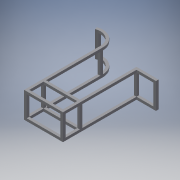
# Autodesk Inventor part: Frame
Saved by Autodesk Inventor 2017 (Build 210142000, 142)
## iProperties
Created: 2017-02-13
Part Number: Frame
Material: Generic
Document SubType Name: Modeling
Designer: Koen
Density: 1 g/cm^3
Appearance: Default
Author: Koen
Autodesk Inventor part; units mm, degrees
ref_plane "YZ Plane" through (0, 0, 0) normal (1, 0, 0) x (0, 1, 0)
ref_plane "XZ Plane" through (0, 0, 0) normal (0, 1, 0) x (-1, 0, 0)
ref_plane "XY Plane" through (0, 0, 0) normal (0, 0, 1) x (1, 0, 0)
sketch "Sketch1" plane through (0, 0, 0) normal (0, 0, 1) x (1, 0, 0)
  line L0 (-300, 150) -> (300, 150)
  line L1 (300, 150) -> (300, -150)
  line L2 (300, -150) -> (-300, -150)
  line L3 (-300, -150) -> (-300, 150)
  line L4 (-300, 150) -> (-260, 150)
  line L5 (-260, 150) -> (-260, 1026.7461)
  line L6 (-260, 1026.7461) -> (-300, 1026.7461)
  line L7 (-300, 1026.7461) -> (-300, 150)
  line L8 (300, 150) -> (260, 150)
  line L9 (260, 150) -> (260, 1026.7461)
  line L10 (260, 1026.7461) -> (300, 1026.7461)
  line L11 (300, 1026.7461) -> (300, 150)
  line L12 (300, 1026.7461) -> (600, 1026.7461)
  line L13 (600, 1026.7461) -> (600, 986.7461)
  line L14 (600, 986.7461) -> (300, 986.7461)
  line L15 (300, 986.7461) -> (300, 1026.7461)
  line L16 (-260, 110) -> (260, 110)
  line L17 (260, 110) -> (260, -110)
  line L18 (260, -110) -> (-260, -110)
  line L19 (-260, -110) -> (-260, 110)
  arc A0 (-260, 1026.7461) -> (-578.8395, 1250) centre (-497.5818, 1026.7461) ccw
  arc A1 (-300, 1026.7461) -> (-565.1587, 1212.4123) centre (-497.5818, 1026.7461) ccw
  line L20 (-565.1587, 1212.4123) -> (-578.8395, 1250)
  point P0 (0, 0)
  point P1 (0, 110)
  point P2 (-260, 0)
  dimension "d0" = 40
  dimension "d1" = 40
  dimension "d2" = 40
  dimension "d3" = 40
  dimension "d4" = 40
  dimension "d6" = 600
  dimension "d7" = 1400
  dimension "d8" = 1136.7461
  dimension "d9" = 300
  dimension "d10" = 300
  dimension "d11" = 110
  constraints: 42 end point, 9 parallel, 6 horizontal, 5 perpendicular, 4 point on circle, 3 vertical alignment, 2 centre point, 2 horizontal alignment, 2 midpoint, 2 point on line, 1 coincident, 1 line through centre
  measures "d0" distance between parallel lines of L3 L19
  measures "d1" distance between parallel lines of L2 L18
  measures "d2" distance between parallel lines of L1 L17
  measures "d3" distance between parallel lines of L16 L0
  measures "d4" distance between parallel lines of L12 L14
  measures "d6" distance of L1.end L2.end
  measures "d7" vertical distance of L2.end L20.end
  measures "d8" vertical distance of L1.end L13.end
  measures "d9" distance between parallel lines of L2 L0
  measures "d10" distance of L10.end L12.end
  measures "d11" angle of L6 L20
extrude "Extrusion1" add sketch "Sketch1" along normal mid plane 400
sketch "Sketch2" plane through (-300, -150, 200) normal (0, -1, 0) x (1, 0, 0)
  line L0 (40, 0) -> (40, -400) projected
  line L1 (560, 0) -> (560, -400) projected
  line L2 (600, -400) -> (600, 0) projected
  line L3 (0, 0) -> (600, 0) projected
  line L4 (600, -400) -> (0, -400) projected
  line L5 (0, -400) -> (0, 0) projected
  line L6 (-265.1587, 0) -> (0, 0) projected
  line L7 (0, -400) -> (-265.1587, -400) projected
  line L8 (-265.1587, -400) -> (-265.1587, 0) projected
  line L9 (600, 0) -> (900, 0) projected
  line L10 (900, -400) -> (900, 0) projected
  line L11 (900, -400) -> (600, -400) projected
  line L12 (0, -400) -> (0, 0) projected
  line L13 (-225.1587, -40) -> (0, -40)
  line L14 (0, -40) -> (0, -360)
  line L15 (0, -360) -> (-225.1587, -360)
  line L16 (-225.1587, -360) -> (-225.1587, -40)
  line L17 (560, -400) -> (560, 0) projected
  line L18 (40, -40) -> (560, -40)
  line L19 (560, -40) -> (560, -360)
  line L20 (560, -360) -> (40, -360)
  line L21 (40, -360) -> (40, -40)
  line L22 (600, -40) -> (860, -40)
  line L23 (860, -40) -> (860, -360)
  line L24 (860, -360) -> (600, -360)
  line L25 (600, -360) -> (600, -40)
  point P0 (300, -200)
  point P1 (-225.1587, -200)
  dimension "d14" = 40
  dimension "d15" = 40
  dimension "d16" = 40
  dimension "d17" = 40
  dimension "d18" = 40
  dimension "d19" = 40
  constraints: 24 end point, 6 parallel, 5 point on line, 3 horizontal, 3 perpendicular, 1 horizontal alignment, 1 midpoint
  measures "d14" distance between parallel lines of L6 L13
  measures "d15" distance between parallel lines of L8 L16
  measures "d16" distance between parallel lines of L4 L20
  measures "d17" distance between parallel lines of L11 L24
  measures "d18" distance between parallel lines of L10 L23
  measures "d19" distance between parallel lines of L9 L22
extrude "Extrusion2" cut sketch "Sketch2" against normal through all contours L18 L1 L20 L0 | L5 L15 L16 L13 | L22 L23 L24 L2
sketch "Sketch3" plane through (300, -150, -200) normal (1, 0, 0) x (0, 0, -1)
  line L0 (0, 1136.7461) -> (-400, 1136.7461) projected
  line L1 (-400, 0) -> (-400, 1136.7461) projected
  line L2 (0, 1136.7461) -> (0, 0) projected
  line L3 (0, 0) -> (-400, 0) projected
  line L4 (-360, 260) -> (-400, 260) projected
  line L5 (0, 260) -> (-40, 260) projected
  line L6 (-400, 40) -> (-360, 40) projected
  line L7 (-40, 40) -> (0, 40) projected
  line L8 (0, 1176.7461) -> (-400, 1176.7461) projected
  line L9 (-40, 1308.68) -> (-360, 1308.68) projected
  line L10 (-40, 1372.394) -> (-360, 1372.394) projected
  line L11 (-360, 260) -> (-40, 260)
  line L12 (-40, 260) -> (-40, 40)
  line L13 (-40, 40) -> (-360, 40)
  line L14 (-360, 40) -> (-360, 260)
  line L15 (-360, 300) -> (-400, 300) projected
  line L16 (-360, 1136.7461) -> (-40, 1136.7461)
  line L17 (-40, 1136.7461) -> (-40, 300)
  line L18 (-40, 300) -> (-360, 300)
  line L19 (-360, 300) -> (-360, 1136.7461)
  line L20 (0, 1176.7461) -> (-400, 1176.7461) projected
  line L21 (-40, 1308.68) -> (-40, 1414.3279) projected
  line L22 (-360, 1176.7461) -> (-40, 1176.7461)
  line L23 (-40, 1176.7461) -> (-40, 1337.0311)
  line L24 (-40, 1337.0311) -> (-360, 1337.0311)
  line L25 (-360, 1337.0311) -> (-360, 1176.7461)
  point P0 (-200, 150)
  point P1 (-200, 260)
  point P2 (-360, 150)
  point P3 (-380, 260)
  point P4 (-200, 300)
  point P5 (-40, 1412.722)
  dimension "d22" = 40
  dimension "d23" = 40
  dimension "d24" = 160.2849
  constraints: 24 end point, 6 parallel, 4 midpoint, 3 collinear, 3 horizontal, 3 perpendicular, 2 horizontal alignment, 2 point on line, 2 vertical alignment
  measures "d22" distance between parallel lines of L2 L12
  measures "d23" distance between parallel lines of L2 L17
  measures "d24" distance between parallel lines of L8 L24
extrude "Extrusion3" cut sketch "Sketch3" against normal through all contours L17 L18 L19 L0 | L12 L13 L14 L11 | L8 L25 L9 L23 | L9 L25 L24 L21
body "Solid1"
